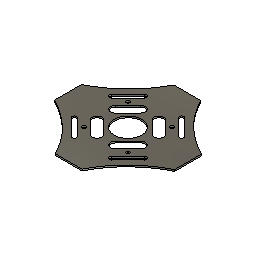
f450 Top (Autodesk Fusion 360 design; units mm, degrees)
Autodesk Fusion 360 part; units mm, degrees
sketch "Sketch1" plane through (0, 0, 0) normal (0, 0, 1) x (1, 0, 0)
  line L0 (-62.25, 0) -> (62.25, 0)
  line L1 (0, -61.5) -> (0, 61.5)
  line L2 (62.25, 0) -> (62.25, 14.0114)
  line L3 (0, 61.5) -> (14.0114, 61.5)
  line L4 (0, -61.5) -> (14.0114, -61.5)
  line L5 (62.25, 0) -> (62.25, -14.0114)
  line L6 (0, 61.5) -> (-14.0114, 61.5)
  line L7 (-62.25, 0) -> (-62.25, 14.0114)
  line L8 (-62.25, 0) -> (-62.25, -14.0114)
  line L9 (0, -61.5) -> (-14.0114, -61.5)
  spline S0 degree 5 poles (62.25, 14.0114) (59.637, 15.2936) (54.5731, 17.9852) (47.4634, 22.4034) (38.8529, 28.9947) (29.2712, 38.3205) (22.5051, 46.7696) (18.0097, 53.821) (15.2968, 58.8805) (14.0114, 61.5) knots 0 0 0 0 0 0 0.2 0.4 0.6 0.8 1 1 1 1 1 1
  line L10 (69.0134, 10.8094) -> (55.9866, 17.2018)
  line L11 (17.2018, 54.9866) -> (10.8094, 68.0134)
  spline S1 degree 5 poles (62.25, -14.0114) (59.637, -15.2936) (54.5731, -17.9852) (47.4634, -22.4034) (38.8529, -28.9947) (29.2712, -38.3205) (22.5051, -46.7696) (18.0097, -53.821) (15.2968, -58.8805) (14.0114, -61.5) knots 0 0 0 0 0 0 0.2 0.4 0.6 0.8 1 1 1 1 1 1
  line L12 (69.0134, -10.8094) -> (55.9866, -17.2018)
  line L13 (17.2018, -54.9866) -> (10.8094, -68.0134)
  spline S2 degree 5 poles (-62.25, -14.0114) (-59.637, -15.2936) (-54.5731, -17.9852) (-47.4634, -22.4034) (-38.8529, -28.9947) (-29.2712, -38.3205) (-22.5051, -46.7696) (-18.0097, -53.821) (-15.2968, -58.8805) (-14.0114, -61.5) knots 0 0 0 0 0 0 0.2 0.4 0.6 0.8 1 1 1 1 1 1
  line L14 (-69.0134, -10.8094) -> (-55.9866, -17.2018)
  line L15 (-17.2018, -54.9866) -> (-10.8094, -68.0134)
  arc A0 (-62.25, 14.0114) -> (-14.0114, 61.5) centre (-113.0267, 113.8346) ccw
  dimension "d1" = 124.5
  dimension "d2" = 123
  constraint horizontal L0
  constraint midpoint origin L0
  constraint perpendicular L0 L1
  constraint midpoint origin L1
  constraint perpendicular L0 L2
  constraint perpendicular L1 L3
  constraint equal L2 L3
  constraint symmetric L0 L11.end L13.end
  measures "d1" distance of L0.start L0.end
  measures "d2" distance of L1.start L1.end
extrude "Extrude1" add sketch "Sketch1" along normal blind 1.6 makes body 1
sketch "Sketch2" plane through (0, 0, 1.6) normal (0, 0, 1) x (-1, 0, 0)
  line L0 (62.25, -14.0114) -> (62.25, 14.0114)
  spline S0 degree 5 poles (62.25, 14.0114) (59.637, 15.2936) (54.5731, 17.9852) (47.4634, 22.4034) (38.8529, 28.9947) (29.2712, 38.3205) (22.5051, 46.7696) (18.0097, 53.821) (15.2968, 58.8805) (14.0114, 61.5) knots 0 0 0 0 0 0 0.2 0.4 0.6 0.8 1 1 1 1 1 1
  line L1 (14.0114, 61.5) -> (-14.0114, 61.5)
  spline S1 degree 5 poles (-14.0114, 61.5) (-15.2968, 58.8805) (-18.0097, 53.821) (-22.5051, 46.7696) (-29.2712, 38.3205) (-38.8529, 28.9947) (-47.4634, 22.4034) (-54.5731, 17.9852) (-59.637, 15.2936) (-62.25, 14.0114) knots -1 -1 -1 -1 -1 -1 -0.8 -0.6 -0.4 -0.2 0 0 0 0 0 0
  line L2 (-62.25, 14.0114) -> (-62.25, -14.0114)
  spline S2 degree 5 poles (-62.25, -14.0114) (-59.637, -15.2936) (-54.5731, -17.9852) (-47.4634, -22.4034) (-38.8529, -28.9947) (-29.2712, -38.3205) (-22.5051, -46.7696) (-18.0097, -53.821) (-15.2968, -58.8805) (-14.0114, -61.5) knots 0 0 0 0 0 0 0.2 0.4 0.6 0.8 1 1 1 1 1 1
  line L3 (-14.0114, -61.5) -> (14.0114, -61.5)
  arc A0 (62.25, -14.0114) -> (14.0114, -61.5) centre (113.0267, -113.8346) ccw
  line L4 (0, -61.5) -> (0, 61.5)
  line L5 (-62.25, 0) -> (62.25, 0)
  line L6 (0, 0) -> (48.1659, 0) construction
  line L7 (0, 0) -> (48.1659, 0) construction
  circle A1 centre (-22.7594, -22.7565) radius 1.9
  circle A2 centre (-0.1033, 0.1166) radius 14.225
  line L8 (-10.0525, -10.0502) -> (-12.6326, -12.632) construction
  line L9 (-12.6326, -12.632) -> (-19.3509, -19.3487) construction
  line L10 (-15.9917, -15.9904) -> (-5.9873, -25.9971) construction
  line L11 (-5.9865, -19.1768) -> (-19.1759, -5.9844)
  arc A3 (-19.1759, -5.9844) -> (-25.9969, -12.8039) centre (-22.5864, -9.3942) ccw
  line L12 (-25.9969, -12.8039) -> (-12.8076, -25.9963)
  arc A4 (-12.8076, -25.9963) -> (-5.9865, -19.1768) centre (-9.3971, -22.5866) ccw
  line L13 (-5.9873, -25.9971) -> (-25.9961, -5.9836) construction
  line L14 (-29.5504, -29.5459) -> (-26.0125, -26.0088) construction
  line L15 (-27.7814, -27.7773) -> (-17.7764, -37.7834) construction
  line L16 (-17.7762, -34.4238) -> (-34.4269, -17.7714)
  arc A5 (-34.4269, -17.7714) -> (-37.7867, -21.1309) centre (-36.1068, -19.4511) ccw
  line L17 (-37.7867, -21.1309) -> (-21.136, -37.7832)
  arc A6 (-21.136, -37.7832) -> (-17.7762, -34.4238) centre (-19.4561, -36.1035) ccw
  line L18 (-17.7764, -37.7834) -> (-37.7865, -17.7713) construction
  line L19 (25.9969, -12.8039) -> (12.8076, -25.9963)
  line L20 (5.9865, -19.1768) -> (19.1759, -5.9844)
  arc A7 (5.9865, -19.1768) -> (12.8076, -25.9963) centre (9.3971, -22.5866) ccw
  arc A8 (25.9969, -12.8039) -> (19.1759, -5.9844) centre (22.5864, -9.3942) ccw
  circle A9 centre (22.7594, -22.7565) radius 1.9
  line L21 (17.7762, -34.4238) -> (34.4269, -17.7714)
  line L22 (37.7867, -21.1309) -> (21.136, -37.7832)
  arc A10 (17.7762, -34.4238) -> (21.136, -37.7832) centre (19.4561, -36.1035) ccw
  arc A11 (37.7867, -21.1309) -> (34.4269, -17.7714) centre (36.1068, -19.4511) ccw
  line L23 (37.7867, 21.1309) -> (21.136, 37.7832)
  line L24 (17.7762, 34.4238) -> (34.4269, 17.7714)
  line L25 (25.9969, 12.8039) -> (12.8076, 25.9963)
  arc A12 (19.1759, 5.9844) -> (25.9969, 12.8039) centre (22.5864, 9.3942) ccw
  line L26 (5.9865, 19.1768) -> (19.1759, 5.9844)
  arc A13 (12.8076, 25.9963) -> (5.9865, 19.1768) centre (9.3971, 22.5866) ccw
  arc A14 (21.136, 37.7832) -> (17.7762, 34.4238) centre (19.4561, 36.1035) ccw
  circle A15 centre (22.7594, 22.7565) radius 1.9
  arc A16 (-5.9865, 19.1768) -> (-12.8076, 25.9963) centre (-9.3971, 22.5866) ccw
  line L27 (-25.9969, 12.8039) -> (-12.8076, 25.9963)
  line L28 (-5.9865, 19.1768) -> (-19.1759, 5.9844)
  arc A17 (-25.9969, 12.8039) -> (-19.1759, 5.9844) centre (-22.5864, 9.3942) ccw
  line L29 (-17.7762, 34.4238) -> (-34.4269, 17.7714)
  line L30 (-37.7867, 21.1309) -> (-21.136, 37.7832)
  arc A18 (-17.7762, 34.4238) -> (-21.136, 37.7832) centre (-19.4561, 36.1035) ccw
  arc A19 (-37.7867, 21.1309) -> (-34.4269, 17.7714) centre (-36.1068, 19.4511) ccw
  circle A20 centre (-22.7594, 22.7565) radius 1.9
  arc A21 (34.4269, 17.7714) -> (37.7867, 21.1309) centre (36.1068, 19.4511) ccw
  line L31 (0, 0) -> (44.5411, 0) construction
  line L32 (0, 0) -> (-10.0513, -10.0513)
  line L33 (0, 0) -> (14.225, 0) construction
  point P0 (-12.6326, -12.632)
  point P1 (-19.3509, -19.3487)
  point P2 (-24.1031, -24.0998)
  point P3 (-21.4158, -21.4131)
  point P4 (-29.5504, -29.5459)
  point P5 (-26.0125, -26.0088)
  point P6 (36.1068, 19.4511)
  point P7 (-27.7814, -27.7773)
  dimension "d10" = 3.8
  dimension "d12" = 28.45
  dimension "d13" = 3.65
  dimension "d14" = 9.5
  dimension "d18" = 28.3
  dimension "d19" = 2.9198
  dimension "d21" = 2.7
  dimension "d24" = 28.3
  dimension "d29" = 135
  constraint midpoint L3 L4.start
  constraint midpoint L1 L4.end
  constraint midpoint L2 L5.start
  constraint midpoint L0 L5.end
  constraint horizontal L6
  constraint coincident L6.start L7.start
  constraint horizontal L7
  constraint coincident A2 L8.start
  constraint coincident P0 L8.end
  constraint coincident A1 P2
  constraint coincident P1 L9.end
  constraint midpoint L9 L10.start
  constraint tangent L11 A3
  constraint tangent A3 L12
  constraint parallel L11 L12
  constraint tangent L12 A4
  constraint tangent L11 A4
  constraint midpoint L10.end A4
  constraint midpoint A3 L13.end
  constraint perpendicular L9 L13
  constraint coincident A1 P3
  constraint coincident P4 L14.start
  constraint coincident P5 L14.end
  constraint midpoint L14 P7
  constraint tangent L16 A5
  constraint tangent A5 L17
  constraint parallel L16 L17
  constraint tangent L17 A6
  constraint tangent L16 A6
  constraint midpoint L15.end A6
  constraint midpoint A5 L18.end
  constraint midpoint L10.start L13
  constraint midpoint P7 L18
  constraint symmetric L4 A1 A9
  constraint symmetric L4 L11.start L20.start
  constraint symmetric L4 L11.end L20.end
  constraint symmetric L4 A3.end L19.start
  constraint symmetric L4 L12.end L19.end
  constraint symmetric L4 A3 A8
  constraint symmetric L4 A4 A7
  constraint symmetric L4 L16.start L21.start
  constraint symmetric L4 L16.end L21.end
  constraint symmetric L4 A5.end L22.start
  constraint symmetric L4 L17.end L22.end
  constraint symmetric L4 A5 A11
  constraint symmetric L4 A6 A10
  constraint symmetric L5 A1 A20
  constraint symmetric L5 L11.start A16.start
  constraint symmetric L5 L11.end L28.end
  constraint symmetric L5 A3.end L27.start
  constraint symmetric L5 L12.end A16.end
  constraint symmetric L5 A3 A17
  constraint symmetric L5 A4 A16
  constraint symmetric L5 L16.start L29.start
  constraint symmetric L5 L16.end L29.end
  constraint symmetric L5 A5.end L30.start
  constraint symmetric L5 L17.end L30.end
  constraint symmetric L5 A5 A19
  constraint symmetric L5 A6 A18
  constraint symmetric L5 L19.start L25.start
  constraint symmetric L5 L19.end L25.end
  constraint symmetric L5 L20.start L26.start
  constraint symmetric L5 L20.end A12.start
  constraint symmetric L5 A7 A13
  constraint symmetric L5 A8 A12
  constraint symmetric L5 A9 A15
  constraint symmetric L5 L21.start L24.start
  constraint symmetric L5 L21.end L24.end
  constraint symmetric L5 L22.start L23.start
  constraint symmetric L5 L22.end L23.end
  constraint symmetric L5 A10 A14
  constraint symmetric L5 A11.centre P6
  constraint symmetric L7 L21.end L24.end
  constraint symmetric L7 L22.start L23.start
  constraint symmetric L7 A11 A21
  constraint horizontal L31
  constraint coincident P7 L15.start
  constraint horizontal L33
  constraint coincident A2 L32.end
  constraint collinear P2 P4 P5
  constraint collinear P2 P3 P5
  constraint collinear P1 P2 P3
  constraint collinear P0 P1 P3
  constraint collinear P0 P1 L32.end
  measures "d10" diameter of A1
  measures "d12" diameter of A2
  measures "d13" distance of L8.start P0
  measures "d14" distance of P0 P1
  measures "d18" distance of L10.end L13.end
  measures "d19" distance of P1 P3
  measures "d21" distance of P2 P5
  measures "d24" distance of L15.end L18.end
  measures "d29" angle of L32 L33
extrude "Extrude2" cut sketch "Sketch2" against normal blind 50 contours L4 L5 A2 | L4 L5 A2 | L4 L5 A2 | L5 A2 L32 | L4 A2 L32 | A1 | L11 A3 L12 A4 | L16 A5 L17 A6 | L19 L20 A7 A8 | A9 | L21 L22 A10 A11 | L23 L24 A14 A21 | L25 A12 L26 A13 | A15 | A16 L27 L28 A17 | L29 L30 A18 A19 | A20 bodies 1
copy_body "Body->Comp1" bodies 1 removing the originals makes body 2 in component "Frame Top"
component "Frame Top" placed x (1, 0, 0) y (0, 1, 0) z (0, 0, 1) at (0, 0, 0)
